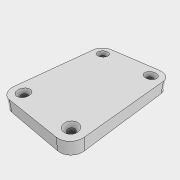
# Autodesk Inventor part: Base plate
Saved by Autodesk Inventor 2020.1 (Build 241239000, 239)
## iProperties
Created: 2019-10-07
Part Number: Base plate
Material: Generic
Document SubType Name: Modeling
Designer: thom_tremblay
Density: 1 g/cm^3
Appearance: Default
Author: thom_tremblay
Autodesk Inventor part; units mm, degrees
ref_plane "YZ Plane" through (0, 0, 0) normal (1, 0, 0) x (0, 1, 0)
ref_plane "XZ Plane" through (0, 0, 0) normal (0, 1, 0) x (-1, 0, 0)
ref_plane "XY Plane" through (0, 0, 0) normal (0, 0, 1) x (1, 0, 0)
sketch "Sketch1" plane through (0, 0, 0) normal (0, 1, 0) x (-1, 0, 0)
  line L0 (-40.64, 58.42) -> (40.64, 58.42)
  line L1 (40.64, 58.42) -> (40.64, -58.42)
  line L2 (40.64, -58.42) -> (-40.64, -58.42)
  line L3 (-40.64, -58.42) -> (-40.64, 58.42)
  point P0 (0, 0)
  point P1 (0, 58.42)
  point P2 (40.64, 0)
  dimension "d0" = 81.28
  dimension "d1" = 116.84
  constraints: 8 end point, 2 midpoint, 2 parallel, 1 horizontal, 1 horizontal alignment, 1 perpendicular, 1 vertical alignment
  measures "d0" distance of L1.end L2.end
  measures "d1" distance of L0.end L1.end
extrude "Extrusion1" add sketch "Sketch1" along normal blind 12.7
fillet "Fillet1" radius 12.7 4 edges at (-40.64, 6.35, 58.42) (-40.64, 6.35, -58.42) (40.64, 6.35, 58.42) (40.64, 6.35, -58.42)
sketch "Sketch2" plane through (0, 12.7, 0) normal (0, 1, 0) x (1, 0, 0)
  arc A0 (-27.94, 58.42) -> (-40.64, 45.72) centre (-27.94, 45.72) ccw projected
  point P0 (0, 0)
  constraints: 1 coincident
hole "Hole1" at (-27.94, 12.7, -45.72) direction (0, -1, 0) diameter 6.7564 end through all countersink diameter 12.8778 countersink angle 82 clearance for "Flat Head Machine Screw (82)" size "1/4" standard "Ansi Unified Screw Threads"
sketch "Sketch3" plane through (0, 12.7, 0) normal (0, 1, 0) x (1, 0, 0)
  arc A0 (-40.64, -45.72) -> (-27.94, -58.42) centre (-27.94, -45.72) ccw projected
  point P0 (0, 0)
  constraints: 1 coincident
hole "Hole2" at (-27.94, 12.7, 45.72) direction (0, -1, 0) diameter 6.7564 end through all countersink diameter 12.8778 countersink angle 82 clearance for "Flat Head Machine Screw (82)" size "1/4" standard "Ansi Unified Screw Threads"
sketch "Sketch4" plane through (0, 12.7, 0) normal (0, 1, 0) x (1, 0, 0)
  arc A0 (27.94, -58.42) -> (40.64, -45.72) centre (27.94, -45.72) ccw projected
  point P0 (0, 0)
  constraints: 1 coincident
hole "Hole3" at (27.94, 12.7, 45.72) direction (0, -1, 0) diameter 6.7564 end through all countersink diameter 12.8778 countersink angle 82 clearance for "Flat Head Machine Screw (82)" size "1/4" standard "Ansi Unified Screw Threads"
sketch "Sketch5" plane through (0, 12.7, 0) normal (0, 1, 0) x (1, 0, 0)
  arc A0 (40.64, 45.72) -> (27.94, 58.42) centre (27.94, 45.72) ccw projected
  point P0 (0, 0)
  constraints: 1 coincident
hole "Hole4" at (27.94, 12.7, -45.72) direction (0, -1, 0) diameter 6.7564 end through all countersink diameter 12.8778 countersink angle 82 clearance for "Flat Head Machine Screw (82)" size "1/4" standard "Ansi Unified Screw Threads"
body "Solid1"
